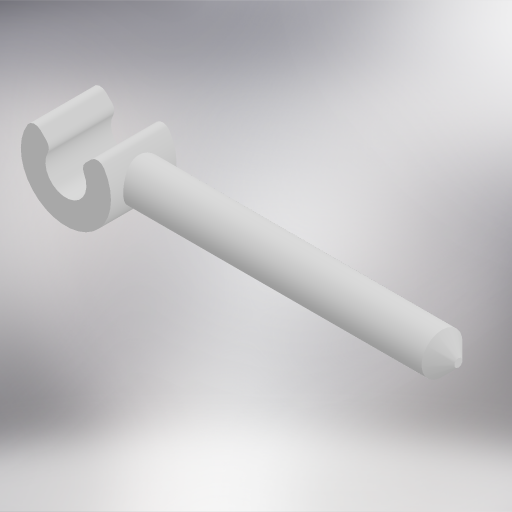
# Autodesk Inventor part: Apple_logo_Black_Part2
Saved by Autodesk Inventor 2024 (Build 280153000, 153)
## iProperties
Created: 2023-10-30
Part Number: Apple_logo_Black_Part2
Material: Generic
Document SubType Name: Modeling
Designer: SSAFY
Density: 1 g/cm^3
Appearance: Default
Author: SSAFY
Autodesk Inventor part; units mm, degrees
ref_plane "YZ Plane" through (0, 0, 0) normal (1, 0, 0) x (0, 1, 0)
ref_plane "XZ Plane" through (0, 0, 0) normal (0, 1, 0) x (-1, 0, 0)
ref_plane "XY Plane" through (0, 0, 0) normal (0, 0, 1) x (1, 0, 0)
sketch "Sketch1" plane through (0, 0, 0) normal (0, 0, 1) x (1, 0, 0)
  circle A0 centre (0, 0) radius 5.5
  circle A1 centre (0, 0) radius 2.5
  line L0 (0, 0) -> (0, 5.5) construction
  line L1 (0, 0) -> (-3.8891, 3.8891)
  line L2 (0, 0) -> (3.8891, 3.8891)
  point P0 (1.7678, 1.7678)
  point P1 (-1.7678, 1.7678)
  dimension "d0" = 5
  dimension "d1" = 3
  dimension "d2" = 45
  dimension "d3" = 45
  constraints: 6 end point, 3 point on circle, 2 centre point, 2 coincident, 1 vertical
  measures "d0" diameter of A1
  measures "d1" radial gap between concentric circles of A0 A1
  measures "d2" angle of L0 L1
  measures "d3" angle of L2 L0
extrude "Extrusion1" add sketch "Sketch1" along normal mid plane 8 contours A0 L1 A1 L2 picked at (-3.4581, 2.8281)
sketch "Sketch2" plane through (0, 0, 0) normal (0, 0, 1) x (1, 0, 0)
  arc A0 (-3.8891, 3.8891) -> (3.8891, 3.8891) centre (0, 0) ccw construction
  line L0 (4.899, 2.5) -> (43.899, 2.5)
  line L1 (43.899, 2.5) -> (43.899, -2.5)
  line L2 (43.899, -2.5) -> (4.899, -2.5)
  line L3 (4.899, -2.5) -> (4.899, 2.5)
  line L4 (0, 0) -> (43.899, 0)
  point P0 (4.899, 0)
  dimension "d6" = 39
  dimension "d7" = 5
  constraints: 10 end point, 2 parallel, 2 point on circle, 1 horizontal, 1 midpoint, 1 perpendicular
  measures "d6" distance of L0.start L0.end
  measures "d7" distance of L0.end L1.end
revolve "Revolution1" add sketch "Sketch2" angle 360 about axis through (0, 0, 0) along (1, 0, 0) contours L0 L1 L4 L3
chamfer "Chamfer1" distance 2 angle 45 1 edges at (43.899, -2.5, 0)
fillet "Fillet3" radius 1 4 edges at (-3.8891, 3.8891, 0) (-1.7678, 1.7678, 0) (3.8891, 3.8891, 0) (1.7678, 1.7678, 0)
body "Solid1"
